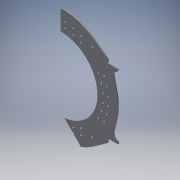
# Autodesk Inventor part: 13in outer coil
Saved by Autodesk Inventor 2016 (Build 200138000, 138)
## iProperties
Created: 2016-02-03
Part Number: 13in outer coil
Material: Generic
Document SubType Name: Modeling
Designer: Scott
Density: 1 g/cm^3
Appearance: Default
Author: Scott
Autodesk Inventor part; units mm, degrees
ref_plane "YZ Plane" through (0, 0, 0) normal (1, 0, 0) x (0, 1, 0)
ref_plane "XZ Plane" through (0, 0, 0) normal (0, 1, 0) x (-1, 0, 0)
ref_plane "XY Plane" through (0, 0, 0) normal (0, 0, 1) x (1, 0, 0)
sketch "Sketch1" plane through (0, 0, 0) normal (0, 0, 1) x (1, 0, 0)
  circle A0 centre (146.7716, -66.8928) radius 3.302 projected
  circle A1 centre (142.4086, -41.8704) radius 3.302 projected
  circle A2 centre (115.6509, -18.469) radius 3.302 projected
  circle A3 centre (12.7, 67.1787) radius 3.302 projected
  circle A4 centre (37.7225, 62.8157) radius 3.302 projected
  circle A5 centre (61.6236, 54.2194) radius 3.302 projected
  circle A6 centre (-37.6212, 45.6905) radius 3.302 projected
  circle A7 centre (-12.7, 67.1787) radius 3.302 projected
  circle A8 centre (-61.6236, 54.2194) radius 3.302 projected
  circle A9 centre (-133.8122, -17.9693) radius 3.302 projected
  circle A10 centre (-130.192, -66.8928) radius 3.302 projected
  circle A11 centre (-146.7716, -66.8928) radius 3.302 projected
  circle A12 centre (-142.4086, -41.8704) radius 3.302 projected
  circle A13 centre (-125.2833, -41.9717) radius 3.302 projected
  circle A14 centre (-115.6509, -18.469) radius 3.302 projected
  circle A15 centre (-37.7225, 62.8157) radius 3.302 projected
  circle A16 centre (-12.7, 50.5992) radius 3.302 projected
  circle A17 centre (-61.1239, 36.0581) radius 3.302 projected
  circle A18 centre (61.1239, 36.0581) radius 3.302 projected
  circle A19 centre (37.6212, 45.6905) radius 3.302 projected
  circle A20 centre (12.7, 50.5992) radius 3.302 projected
  circle A21 centre (133.8122, -17.9693) radius 3.302 projected
  circle A22 centre (125.2833, -41.9717) radius 3.302 projected
  circle A23 centre (130.192, -66.8928) radius 3.302 projected
  arc A24 (165.1, -79.5928) -> (-165.1, -79.5928) centre (0, -79.5928) ccw projected
  line L0 (-114.3, -79.5928) -> (-165.1, -79.5928) projected
  arc A25 (114.3, -79.5928) -> (-114.3, -79.5928) centre (0, -79.5928) ccw projected
  line L1 (165.1, -79.5928) -> (114.3, -79.5928) projected
  circle A26 centre (-146.7716, -92.2928) radius 3.302 projected
  circle A27 centre (-142.4086, -117.3153) radius 3.302 projected
  circle A28 centre (-115.6509, -140.7167) radius 3.302 projected
  circle A29 centre (-12.7, -226.3644) radius 3.302 projected
  circle A30 centre (-37.7225, -222.0014) radius 3.302 projected
  circle A31 centre (-61.6236, -213.4051) radius 3.302 projected
  circle A32 centre (37.6212, -204.8761) radius 3.302 projected
  circle A33 centre (12.7, -226.3644) radius 3.302 projected
  circle A34 centre (61.6236, -213.4051) radius 3.302 projected
  circle A35 centre (133.8122, -141.2164) radius 3.302 projected
  circle A36 centre (130.192, -92.2928) radius 3.302 projected
  circle A37 centre (146.7716, -92.2928) radius 3.302 projected
  circle A38 centre (142.4086, -117.3153) radius 3.302 projected
  circle A39 centre (125.2833, -117.214) radius 3.302 projected
  circle A40 centre (115.6509, -140.7167) radius 3.302 projected
  circle A41 centre (37.7225, -222.0014) radius 3.302 projected
  circle A42 centre (12.7, -209.7849) radius 3.302 projected
  circle A43 centre (61.1239, -195.2437) radius 3.302 projected
  circle A44 centre (-61.1239, -195.2437) radius 3.302 projected
  circle A45 centre (-37.6212, -204.8761) radius 3.302 projected
  circle A46 centre (-12.7, -209.7849) radius 3.302 projected
  circle A47 centre (-133.8122, -141.2164) radius 3.302 projected
  circle A48 centre (-125.2833, -117.214) radius 3.302 projected
  circle A49 centre (-130.192, -92.2928) radius 3.302 projected
  arc A50 (-165.1, -79.5928) -> (165.1, -79.5928) centre (0, -79.5928) ccw projected
  line L2 (114.3, -79.5928) -> (165.1, -79.5928) projected
  arc A51 (-114.3, -79.5928) -> (114.3, -79.5928) centre (0, -79.5928) ccw projected
  line L3 (-165.1, -79.5928) -> (-114.3, -79.5928) projected
  arc A52 (0, -257.3928) -> (0, 98.2072) centre (0, -79.5928) ccw
  line L4 (0, 98.2072) -> (0, 34.7072)
  line L5 (0, -193.8928) -> (0, -257.3928)
  point P0 (0, 0)
  dimension "d0" = 355.6
  constraints: 4 end point, 4 point on circle, 2 vertical, 1 centre point, 1 coincident
  measures "d0" diameter of A52
extrude "Extrusion1" add sketch "Sketch1" along normal blind 3.175 contours L1 A25 L4 A24 | A50 L5 A51 L1 | A24 L4 A52 L5 A50
sketch "Sketch2" plane through (0, 0, 0) normal (0, 0, -1) x (-1, 0, 0)
  arc A0 (0, 98.2072) -> (0, -257.3928) centre (0, -79.5928) ccw projected
  line L0 (-215.9, -184.3678) -> (-163.2323, -184.3678) projected
  line L1 (-152.4, -184.3678) -> (0, -184.3678) projected
  line L2 (152.4, -190.7178) -> (-152.4, -190.7178) projected
  line L3 (152.4, -190.7178) -> (-152.4, -190.7178) projected
  line L4 (-215.9, -181.1928) -> (-163.2323, -181.1928) projected
  line L5 (0, -190.7178) -> (-203.2, -190.7178) projected
  line L6 (-46.5518, -181.1928) -> (46.5518, -181.1928) projected
  line L7 (152.4, -181.1928) -> (-152.4, -181.1928) projected
  line L8 (-163.2323, -193.8928) -> (-215.9, -193.8928) projected
  line L9 (0, -184.3678) -> (-203.2, -184.3678) projected
  line L10 (-127, -193.8928) -> (-163.2323, -193.8928) projected
  arc A1 (0, 98.2072) -> (0, -257.3928) centre (0, -79.5928) ccw projected
  line L11 (-145.9119, -181.1928) -> (-145.9119, -193.8928)
  line L12 (-145.9119, -193.8928) -> (-136.1923, -193.8928)
  arc A2 (-145.9119, -181.1928) -> (-136.1923, -193.8928) centre (0, -79.5928) ccw
  line L13 (-145.9119, -181.1928) -> (-158.6119, -181.1928)
  line L14 (-158.6119, -181.1928) -> (-172.9857, -120.6879)
  line L15 (-145.9119, -193.8928) -> (-103.2908, -224.3128)
  arc A3 (-172.9857, -120.6879) -> (-145.9119, -181.1928) centre (0, -79.5928) ccw
  arc A4 (-145.9119, -181.1928) -> (-103.2908, -224.3128) centre (0, -79.5928) ccw
  line L16 (0, -79.5928) -> (-43.5104, -79.5928) construction
  line L17 (-145.9119, 22.0072) -> (-145.9119, 34.7072)
  line L18 (-145.9119, 22.0072) -> (-158.6119, 22.0072)
  line L19 (-158.6119, 22.0072) -> (-172.9857, -38.4978)
  line L20 (-145.9119, 34.7072) -> (-103.2908, 65.1271)
  arc A5 (-145.9119, 22.0072) -> (-172.9857, -38.4978) centre (0, -79.5928) ccw
  arc A6 (-103.2908, 65.1271) -> (-145.9119, 22.0072) centre (0, -79.5928) ccw
  point P0 (0, 0)
  dimension "d3" = 12.7
  constraints: 20 end point, 16 point on circle, 5 centre point, 5 symmetric about line, 4 point on line, 2 tangent, 1 horizontal, 1 perpendicular
  measures "d3" distance of L11.start L13.end
extrude "Extrusion3" add sketch "Sketch2" against normal blind 3.175
sketch "Sketch3" plane through (0, 0, 0) normal (0, 0, -1) x (-1, 0, 0)
  circle A0 centre (-61.1239, -195.2437) radius 3.302 projected
  circle A1 centre (-12.7, -209.7849) radius 3.302 projected
  circle A2 centre (-37.7225, -222.0014) radius 3.302 projected
  circle A3 centre (-115.6509, -140.7167) radius 3.302 projected
  circle A4 centre (-125.2833, -117.214) radius 3.302 projected
  circle A5 centre (-142.4086, -117.3153) radius 3.302 projected
  circle A6 centre (-146.7716, -92.2928) radius 3.302 projected
  circle A7 centre (-130.192, -92.2928) radius 3.302 projected
  circle A8 centre (-133.8122, -141.2164) radius 3.302 projected
  circle A9 centre (-61.6236, -213.4051) radius 3.302 projected
  circle A10 centre (-12.7, -226.3644) radius 3.302 projected
  circle A11 centre (-37.6212, -204.8761) radius 3.302 projected
  circle A12 centre (-130.192, -66.8928) radius 3.302 projected
  circle A13 centre (-125.2833, -41.9717) radius 3.302 projected
  circle A14 centre (-133.8122, -17.9693) radius 3.302 projected
  circle A15 centre (-12.7, 50.5992) radius 3.302 projected
  circle A16 centre (-37.6212, 45.6905) radius 3.302 projected
  circle A17 centre (-61.1239, 36.0581) radius 3.302 projected
  circle A18 centre (-61.6236, 54.2194) radius 3.302 projected
  circle A19 centre (-37.7225, 62.8157) radius 3.302 projected
  circle A20 centre (-12.7, 67.1787) radius 3.302 projected
  circle A21 centre (-115.6509, -18.469) radius 3.302 projected
  circle A22 centre (-142.4086, -41.8704) radius 3.302 projected
  circle A23 centre (-146.7716, -66.8928) radius 3.302 projected
  arc A24 (0, 34.7072) -> (0, -193.8928) centre (0, -79.5928) ccw projected
  line L0 (0, 98.2072) -> (0, 34.7072) projected
  arc A25 (0, 98.2072) -> (-103.2908, 65.1271) centre (0, -79.5928) ccw projected
  line L1 (-103.2908, 65.1271) -> (-145.9119, 34.7072) projected
  line L2 (-145.9119, 34.7072) -> (-145.9119, 22.0072) projected
  line L3 (-145.9119, 22.0072) -> (-158.6119, 22.0072) projected
  line L4 (-158.6119, 22.0072) -> (-172.9857, -38.4978) projected
  arc A26 (-172.9857, -38.4978) -> (-172.9857, -120.6879) centre (0, -79.5928) ccw projected
  line L5 (-172.9857, -120.6879) -> (-158.6119, -181.1928) projected
  line L6 (-158.6119, -181.1928) -> (-145.9119, -181.1928) projected
  line L7 (-145.9119, -181.1928) -> (-145.9119, -193.8928) projected
  line L8 (-145.9119, -193.8928) -> (-103.2908, -224.3128) projected
  arc A27 (-103.2908, -224.3128) -> (0, -257.3928) centre (0, -79.5928) ccw projected
  line L9 (0, -193.8928) -> (0, -257.3928) projected
  line L10 (-145.9119, -181.1928) -> (-158.6119, -181.1928) projected
  line L11 (-158.6119, -181.1928) -> (-178.9319, -181.1928)
  circle A28 centre (0, -79.5928) radius 177.8
  arc A29 (-172.4957, -170.8784) -> (-178.9319, -181.1928) centre (-169.0032, -180.223) ccw
  arc A30 (-172.4957, -170.8784) -> (-164.5857, -156.0467) centre (-176.9418, -158.9821) ccw
  arc A31 (-172.9857, -38.4978) -> (-172.9857, -120.6879) centre (0, -79.5928) ccw projected
  line L12 (0, -79.5928) -> (-220.3249, -79.5928)
  line L13 (-158.6119, -181.1928) -> (-172.9857, -120.6879) projected
  line L14 (-164.5857, -156.0467) -> (-158.6119, -181.1928)
  line L15 (-172.9857, -38.4978) -> (-164.5857, -3.139)
  line L16 (-158.6119, 22.0072) -> (-178.9319, 22.0072)
  arc A32 (-178.9319, 22.0072) -> (-172.4957, 11.6927) centre (-169.0032, 21.0374) ccw
  arc A33 (-164.5857, -3.139) -> (-172.4957, 11.6927) centre (-176.9418, -0.2036) ccw
  line L17 (-164.5857, -3.139) -> (-158.6119, 22.0072)
  point P0 (0, 0)
  point P1 (-159.6945, -176.6356)
  dimension "d8" = 20.32
  dimension "d9" = 12.7
  constraints: 12 end point, 9 point on circle, 5 centre point, 5 symmetric about line, 3 tangent, 2 horizontal, 1 coincident, 1 collinear, 1 point on line, 2 other
  measures "d8" distance of L5.end L11.end
  measures "d9" radius of A30
extrude "Extrusion4" add sketch "Sketch3" against normal blind 3.175 contours A33 A32 L16 L4 | L5 L11 A29 A30
sketch "Sketch4" plane through (0, 0, 3.175) normal (0, 0, 1) x (1, 0, 0)
  circle A0 centre (96.1901, -201.0584) radius 3.302 projected
  circle A1 centre (96.1901, 41.8727) radius 3.302 projected
  point P0 (0, 0)
extrude "Extrusion5" cut sketch "Sketch4" against normal blind 3.175
body "Solid1"
